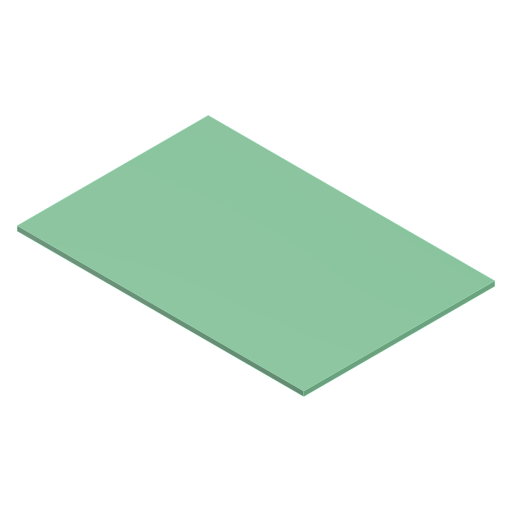
# Autodesk Inventor part: table_kan
Saved by Autodesk Inventor 2023 (Build 270158000, 158)
## iProperties
Created: 2024-12-03
Part Number: table_kan
Material: Generic
Document SubType Name: Modeling
Designer: kiyo
Density: 1 g/cm^3
Appearance: 滑らか - 濃い海緑
Author: kiyo
Autodesk Inventor part; units mm, degrees
ref_plane "YZ Plane" through (0, 0, 0) normal (1, 0, 0) x (0, 1, 0)
ref_plane "XZ Plane" through (0, 0, 0) normal (0, 1, 0) x (-1, 0, 0)
ref_plane "XY Plane" through (0, 0, 0) normal (0, 0, 1) x (1, 0, 0)
sketch "スケッチ1" plane through (0, 0, 0) normal (0, 1, 0) x (-1, 0, 0)
  line L0 (0, 0) -> (-1000, 0)
  line L1 (-1000, 0) -> (-1000, 25)
  line L2 (-1000, 25) -> (0, 25)
  line L3 (0, 25) -> (0, 0)
  dimension "d0" = 25
  dimension "d1" = 1000
  constraints: 8 end point, 2 parallel, 1 horizontal, 1 perpendicular
  measures "d0" distance of L0.end L1.end
  measures "d1" distance of L0.start L0.end
extrude "押し出し1" add sketch "スケッチ1" along normal mid plane 1500
sketch "スケッチ2" plane through (0, -750, 25) normal (0, 0, 1) x (1, 0, 0)
  circle A0 centre (500, 1150) radius 33
  line L0 (0, 1500) -> (0, 750) projected
  line L1 (0, 1500) -> (1000, 1500) projected
  dimension "d4" = 66
  dimension "d6" = 500
  dimension "d10" = 350
  constraints: 1 centre point
  measures "d4" diameter of A0
  measures "d6" distance from line of L0 A0.centre
  measures "d10" distance from line of L1 A0.centre
extrude "押し出し2" [suppressed]
